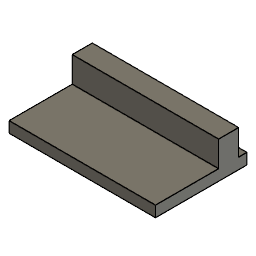
my_test_potok (Autodesk Fusion 360 design; units mm, degrees)
Autodesk Fusion 360 part; units mm, degrees
sketch "Sketch1" plane through (0, 0, 0) normal (0, 1, 0) x (1, 0, 0)
  line L0 (8, -5) -> (-8, -5)
  line L1 (-8, -5) -> (-8, 5)
  line L2 (-8, 5) -> (8, 5)
  line L3 (8, 5) -> (8, -5)
  line L4 (8, -5) -> (-8, 5) construction
  line L5 (-8, -5) -> (8, 5) construction
  line L6 (8, 1.9) -> (-8, 1.9)
  line L7 (-8, 1.9) -> (-8, 4.1)
  line L8 (-8, 4.1) -> (8, 4.1)
  line L9 (8, 4.1) -> (8, 1.9)
  line L10 (8, 1.9) -> (-8, 4.1) construction
  line L11 (-8, 1.9) -> (8, 4.1) construction
  point P0 (0, 3)
  dimension "d1" = 16
  dimension "d2" = 10
  dimension "d3" = 2.2
  constraint horizontal L0
  constraint perpendicular L0 L1
  constraint parallel L0 L2
  constraint parallel L1 L3
  constraint coincident L4 origin
  constraint coincident L5 origin
  constraint horizontal L6
  constraint perpendicular L6 L7
  constraint parallel L6 L8
  constraint parallel L7 L9
  constraint coincident L10 P0
  constraint coincident L11 P0
  measures "d1" distance of L1.end L2.end
  measures "d2" distance of L0.end L1.end
  measures "d3" distance of L6.end L7.end
extrude "Extrude1" add sketch "Sketch1" along normal blind 1.2
extrude "Extrude2" add sketch "Sketch1" along normal blind 4 contours L1 L3 L6 L7 L8 L9
